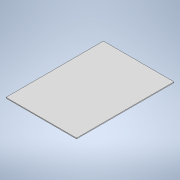
# Autodesk Inventor part: Lift.03.01.00.06
Saved by Autodesk Inventor 2021 (Build 250183000, 183)
## iProperties
Created: 2020-09-20
Part Number: Lift.03.01.00.06
Material: Типовые
Document SubType Name: ЛистМат
Designer: Kostya
Density: 1 g/cm^3
Appearance: По умолчанию
Sheet Metal Rule: По умолчанию_мм
Author: Kostya
Autodesk Inventor part; units mm, degrees
ref_plane "YZ Plane" through (0, 0, 0) normal (1, 0, 0) x (0, 1, 0)
ref_plane "XZ Plane" through (0, 0, 0) normal (0, 1, 0) x (-1, 0, 0)
ref_plane "XY Plane" through (0, 0, 0) normal (0, 0, 1) x (1, 0, 0)
sketch "Эскиз1" plane through (0, 0, 0) normal (0, 1, 0) x (-1, 0, 0)
  line L0 (-900, -1242.5) -> (900, -1242.5)
  line L1 (900, -1242.5) -> (900, 1242.5)
  line L2 (900, 1242.5) -> (-900, 1242.5)
  line L3 (-900, 1242.5) -> (-900, -1242.5)
  line L4 (-900, -1242.5) -> (900, 1242.5) construction
  line L5 (900, -1242.5) -> (-900, 1242.5) construction
  point P0 (0, 0)
  dimension "d0" = 1800
  dimension "d1" = 2485
  measures "d0" distance of L2.end L1.end
  measures "d1" distance of L1.end L0.end
extrude "Пластина1" add sketch "Эскиз1" along normal blind 20
equation "\"d2\" = Толщина"
equation "\"Толщина\" = 20"
